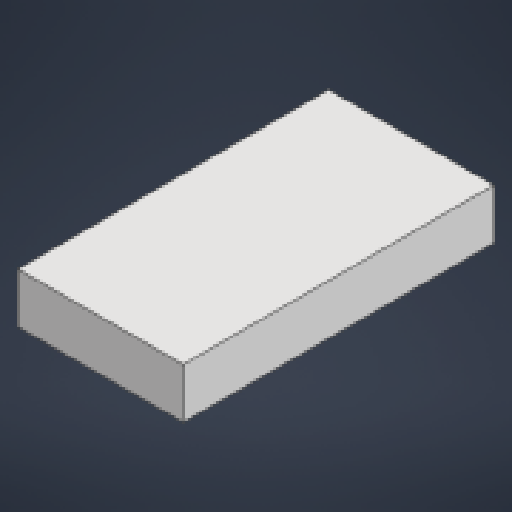
# Autodesk Inventor part: bms
Saved by Autodesk Inventor 2024 (Build 280153000, 153)
## iProperties
Created: 2024-05-06
Part Number: bms
Material: Generic
Document SubType Name: Modeling
Designer: markm
Density: 1 g/cm^3
Appearance: Default
Author: markm
Autodesk Inventor part; units mm, degrees
ref_plane "YZ Plane" through (0, 0, 0) normal (1, 0, 0) x (0, 1, 0)
ref_plane "XZ Plane" through (0, 0, 0) normal (0, 1, 0) x (-1, 0, 0)
ref_plane "XY Plane" through (0, 0, 0) normal (0, 0, 1) x (1, 0, 0)
sketch "Sketch1" plane through (0, 0, 0) normal (0, 1, 0) x (-1, 0, 0)
  line L0 (-16.5, -35) -> (16.5, -35)
  line L1 (16.5, -35) -> (16.5, 35)
  line L2 (16.5, 35) -> (-16.5, 35)
  line L3 (-16.5, 35) -> (-16.5, -35)
  line L4 (-16.5, -35) -> (16.5, 35) construction
  line L5 (16.5, -35) -> (-16.5, 35) construction
  point P0 (0, 0)
  dimension "d0" = 70
  dimension "d1" = 33
  constraints: 12 end point, 2 midpoint, 2 parallel, 1 horizontal, 1 perpendicular
  measures "d0" distance of L1.end L0.end
  measures "d1" distance of L0.start L0.end
extrude "Extrusion1" add sketch "Sketch1" along normal mid plane 10
body "Solid1"
